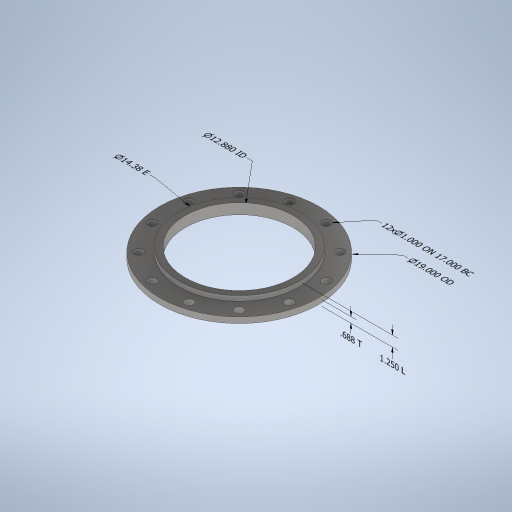
# Autodesk Inventor part: AWWA C207-18 Class B Ring and Blind Flange
Saved by Autodesk Inventor 2023 (Build 270158000, 158)
## iProperties
RuleStatus: InUse
Created: 2023-06-05
Part Number: AWWA C207-18 Class B Ring and Blind Flange
Material: Generic
Document SubType Name: Modeling
Designer: Admin
Density: 1 g/cm^3
Appearance: Steel - Polished
Author: Admin
Autodesk Inventor part; units mm, degrees
ref_plane "YZ Plane" through (0, 0, 0) normal (1, 0, 0) x (0, 1, 0)
ref_plane "XZ Plane" through (0, 0, 0) normal (0, 1, 0) x (-1, 0, 0)
ref_plane "XY Plane" through (0, 0, 0) normal (0, 0, 1) x (1, 0, 0)
sketch "Flange Sketch" plane through (0, 0, 0) normal (0, 1, 0) x (-1, 0, 0)
  circle A0 centre (0, 0) radius 241.3
  circle A1 centre (0, 0) radius 163.576
  circle A2 centre (0, 0) radius 215.9 construction
  line L0 (0, 0) -> (-55.879, -208.5434) construction
  line L1 (0, 0) -> (0, -215.9) construction
  circle A3 centre (0, 0) radius 182.5625
  dimension "outerDiam" = 482.6
  dimension "innerDiam" = 327.152
  dimension "boltCircle" = 431.8
  dimension "boltOffsetAngle" = 15
  dimension "dimensionE" = 365.125
  constraints: 4 centre point, 4 coincident, 4 end point, 2 point on circle, 1 vertical
  measures "outerDiam" diameter of A0
  measures "innerDiam" diameter of A1
  measures "boltCircle" diameter of A2
  measures "boltOffsetAngle" angle of L0 L1
  measures "dimensionE" diameter of A3
extrude "Flange Extrusion" add sketch "Flange Sketch" along normal blind 17.4752 contours A0 | A3
extrude "Flange Exrusion2" add sketch "Flange Sketch" along normal blind 31.75 contours A3
hole "Bolt Hole" at (55.879, 0, -208.5434) direction (0, 1, 0) diameter 25.4 depth 17.4752
pattern_circular "Bolt Hole Pattern" count 12 over 360 about axis through (0, -10, 0) along (0, 1, 0) of "Bolt Hole"
equation "\"nominalSize\" = 304.8"
body "Solid1"
